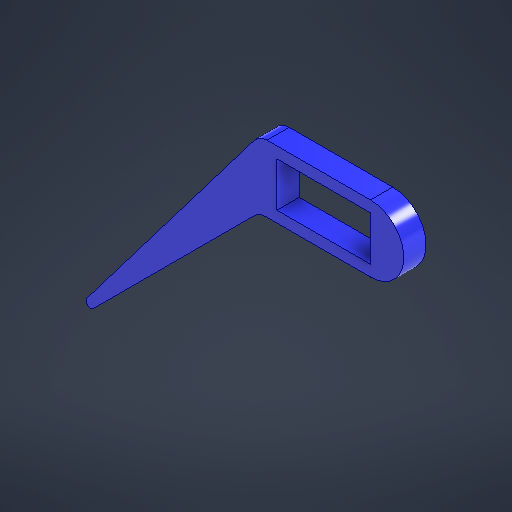
# Autodesk Inventor part: Spider_Robot_Tibia_V1
Saved by Autodesk Inventor 2026.2 (Build 302298010, 298A)
## iProperties
Created: 2026-08-14
Part Number: Spider_Robot_Tibia_V1
Material: Generic
Document SubType Name: Modeling
Designer: Entity
Mass: 23.8297 g
Surface Area: 98.6256 cm^2
Volume: 23.8297 cm^3
Density: 1 g/cm^3
Appearance: Blue - Wall Paint - Glossy
Author: Entity
Autodesk Inventor part; units mm, degrees
ref_plane "YZ Plane" through (0, 0, 0) normal (1, 0, 0) x (0, 1, 0)
ref_plane "XZ Plane" through (0, 0, 0) normal (0, 1, 0) x (-1, 0, 0)
ref_plane "XY Plane" through (0, 0, 0) normal (0, 0, 1) x (1, 0, 0)
sketch "Sketch1" plane through (0, 0, 0) normal (0, 0, 1) x (1, 0, 0)
  line L0 (-21, 10) -> (21, 10)
  line L1 (21, 10) -> (21, -10)
  line L2 (21, -10) -> (-21, -10)
  line L3 (-21, -10) -> (-21, 10)
  arc A0 (21, -15) -> (36, 0) centre (21, 0) ccw
  arc A1 (21, -15) -> (21, 15) centre (21, 0) ccw
  line L4 (21, 15) -> (-25.5259, 15)
  line L5 (21, -15) -> (-26.1005, -15)
  line L6 (-31.0503, -17.0503) -> (-103.2462, -89.2462)
  arc A2 (-106.0355, -86.4569) -> (-103.2462, -89.2462) centre (-104.8753, -88.086) ccw
  line L7 (-106.0355, -86.4569) -> (-31.1009, 12.2331)
  arc A3 (-26.1005, -15) -> (-31.0503, -17.0503) centre (-26.1005, -22) ccw
  arc A4 (-25.5259, 15) -> (-31.1009, 12.2331) centre (-25.5259, 8) ccw
  point P0 (0, 0)
  point P1 (-21, 0)
  point P2 (-29, 15)
  point P3 (-29, -15)
  dimension "d0" = 42
  dimension "d1" = 20
  dimension "d2" = 10
  dimension "d3" = 21
  dimension "d5" = 15
  dimension "d6" = 50
  dimension "d7" = 105
  dimension "d9" = 2
  dimension "d10" = 50
  dimension "d11" = 7
  dimension "d12" = 7
  constraints: 16 end point, 11 point on circle, 5 centre point, 4 point on line, 4 tangent, 3 horizontal, 2 parallel, 1 midpoint, 1 perpendicular
  measures "d0" distance of L0.start L0.end
  measures "d1" distance of L2.end L0.start
  measures "d2" distance from line of L0 point (0, 0)
  measures "d3" distance of point (-21, 0) point (0, 0)
  measures "d5" radius of A1
  measures "d6" distance of L4.start point (-29, 15)
  measures "d7" distance of point (-29, -15) L6.end
  measures "d9" radius of A2
  measures "d10" distance of L5.start point (-29, -15)
  measures "d11" radius of A3
  measures "d12" radius of A4
extrude "Extrusion1" add sketch "Sketch1" along normal blind 10
body "Solid1"
